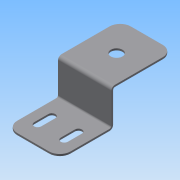
# Autodesk Inventor part: Tunel_IRBeamHolder
Saved by Autodesk Inventor 2016 (Build 200138000, 138)
## iProperties
Created: 2014-11-25
Part Number: Tunel_IRBeamHolder
Material: Generisch
Document SubType Name: Sheet Metal
Designer: Gero Hofmann
Density: 1 g/cm^3
Sheet Metal Rule: Default_mm
Appearance: Vorgabe
Author: Gero Hofmann
Autodesk Inventor part; units mm, degrees
ref_plane "YZ Plane" through (0, 0, 0) normal (1, 0, 0) x (0, 1, 0)
ref_plane "XZ Plane" through (0, 0, 0) normal (0, 1, 0) x (-1, 0, 0)
ref_plane "XY Plane" through (0, 0, 0) normal (0, 0, 1) x (1, 0, 0)
sketch "Skizze1" plane through (0, 0, 0) normal (0, 0, 1) x (1, 0, 0)
  line L0 (-15, 30) -> (15, 30)
  line L1 (15, 30) -> (15, 0)
  line L2 (15, 0) -> (-15, 0)
  line L3 (-15, 0) -> (-15, 30)
  line L4 (-15, 30) -> (15, 0) construction
  line L5 (15, 30) -> (-15, 0) construction
  point P0 (0, 0)
  point P1 (0, 15)
  dimension "d0" = 30
  dimension "d1" = 30
  measures "d0" distance of L1.end L2.end
  measures "d1" distance of L0.end L1.end
extrude "Grobblech1" add sketch "Skizze1" along normal blind 1
sketch "Skizze2" plane through (-15, 29, 0) normal (0, 1, 0) x (-1, 0, 0)
  line L0 (-30, 0) -> (0, 0)
  line L1 (0, 0) -> (0, 21)
  line L2 (0, 21) -> (-30, 21)
  line L3 (-30, 21) -> (-30, 0)
  constraints: 6 end point, 1 horizontal, 1 perpendicular, 1 vertical
edge flange "Lasche1" height 20 angle 90 thickness 1 bend radius 1 thickness toward (0, 1, 0) relief tear relief width 1 relief depth 0.5 edges at (0, 30, 1) wall of the first edge with corners at (15, 29, 0) (-15, 29, 0) (-15, 29, 21) (15, 29, 21)
bend "Biegung1"
corner "Ecke1"
sketch "Skizze3" plane through (15, 29, 20) normal (0, 0, 1) x (1, 0, 0)
  line L0 (-30, 0) -> (0, 0)
  line L1 (0, 0) -> (0, 35)
  line L2 (0, 35) -> (-30, 35)
  line L3 (-30, 35) -> (-30, 0)
  constraints: 6 end point, 1 horizontal, 1 perpendicular, 1 vertical
edge flange "Lasche2" height 34 angle 90 thickness 1 bend radius 1 thickness toward (0, 0, 1) relief tear relief width 1 relief depth 0.5 edges at (0, 30, 21) wall of the first edge with corners at (-15, 29, 20) (15, 29, 20) (15, 64, 20) (-15, 64, 20)
bend "Biegung2"
corner "Ecke2"
hole "Bohrung2" at (0, 47, 21) direction (0, 0, -1) diameter 6.6 end through all clearance for "Sechskantkopfschraube DIN EN 24017" size "M6" standard "DIN"
sketch "Skizze6" plane through (0, 0, 1) normal (0, 0, 1) x (1, 0, 0)
  line L0 (15, 28) -> (-15, 28) projected
  line L1 (-15, 0) -> (-15, 28) projected
  line L2 (7.5, 10) -> (7.5, 18) construction
  line L3 (9.5, 10) -> (9.5, 18)
  line L4 (5.5, 18) -> (5.5, 10)
  arc A0 (5.5, 10) -> (9.5, 10) centre (7.5, 10) ccw
  arc A1 (9.5, 18) -> (5.5, 18) centre (7.5, 18) ccw
  line L5 (0, 28) -> (0, 0) construction
  line L6 (-7.5, 10) -> (-7.5, 18) construction
  line L7 (-9.5, 10) -> (-9.5, 18)
  line L8 (-5.5, 18) -> (-5.5, 10)
  arc A2 (-9.5, 10) -> (-5.5, 10) centre (-7.5, 10) ccw
  arc A3 (-5.5, 18) -> (-9.5, 18) centre (-7.5, 18) ccw
  point P0 (7.5, 14)
  point P1 (-7.5, 14)
  point P2 (0, 14)
  dimension "d47" = 15
  dimension "d48" = 12
  dimension "d50" = 4
  constraints: 18 end point, 8 point on circle, 7 symmetric about line, 4 centre point, 4 tangent, 3 midpoint, 3 parallel, 1 horizontal alignment, 2 other
  measures "d47" distance between parallel lines of L6 L2
  measures "d50" distance between parallel lines of L4 L3
extrude "Extrusion2" cut sketch "Skizze6" against normal through all
fillet "Eckenrundung1" radius 6 4 edges at (15, 0, 0.5) (-15, 0, 0.5) (-15, 64, 20.5) (15, 64, 20.5)
equation "\"d45\" = Stärke"
equation "\"d3\" = BreiteBiegungsfreistellung"
equation "\"d4\" = TiefeBiegungsfreistellung"
equation "\"d5\" = MinimalRest"
equation "\"d6\" = Biegeradius"
equation "\"d9\" = Biegeradius"
equation "\"d10\" = GrößeEckenfreistellung"
equation "\"d11\" = Abstandsgröße"
equation "\"d12\" = JacobiRadiusGröße"
equation "\"d13\" = BreiteBiegungsfreistellung"
equation "\"d14\" = TiefeBiegungsfreistellung"
equation "\"d15\" = MinimalRest"
equation "\"d16\" = Biegeradius"
equation "\"d19\" = Biegeradius"
equation "\"d20\" = GrößeEckenfreistellung"
equation "\"d21\" = Abstandsgröße"
equation "\"d22\" = JacobiRadiusGröße"
equation "\"Biegeradius\" = Stärke"
equation "\"BreiteBiegungsfreistellung\" = Stärke"
equation "\"TiefeBiegungsfreistellung\" = 0.5 * Stärke"
equation "\"GrößeEckenfreistellung\" = 4 * Stärke"
equation "\"MinimalRest\" = 2 * Stärke"
equation "\"Übergangsradius\" = Biegeradius"
equation "\"JacobiRadiusGröße\" = Biegeradius"
equation "\"Abstandsgröße\" = Stärke"
equation "\"d2\" = Biegeradius"
equation "\"Stärke\" = 1"
